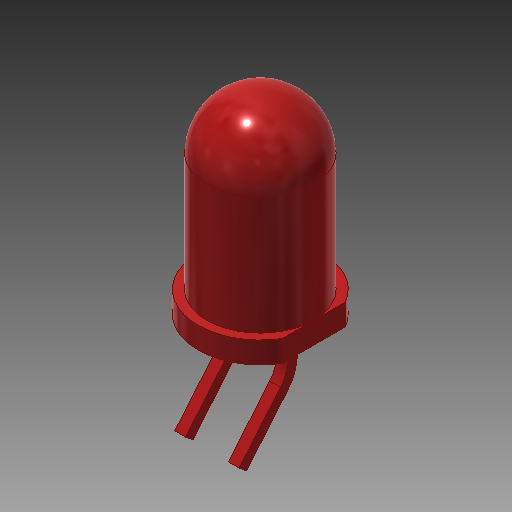
# Autodesk Inventor part: LED 5mm
Saved by Autodesk Inventor 2019.1 (Build 231200000, 200)
## iProperties
Created: 2012-08-15
Part Number: LED 5mm
Material: PC/ABS-Kunststoff
Document SubType Name: Modeling
Designer: rYan
Density: 1.493 g/cm^3
Mass: 0.251814 g
Surface Area: 1.94955 cm^2
Volume: 0.168663 cm^3
Appearance: Hellrot
Author: rYan
Autodesk Inventor part; units mm, degrees
note: some values were not read from the file. Chosen so that the rebuilt part matches the saved one: bend side of "Biegungsteil1".
ref_plane "XZ Plane" through (0, 0, 0) normal (0, 1, 0) x (-1, 0, 0)
ref_plane "XY Plane" through (0, 0, 0) normal (0, 0, 1) x (1, 0, 0)
sketch "Skizze1" plane through (0, 0, 0) normal (0, 1, 0) x (-1, 0, 0)
  line L0 (0, 0) -> (0, 9)
  line L1 (0, 0) -> (2.9, 0)
  line L2 (2.9, 0) -> (2.9, 1)
  line L3 (2.9, 1) -> (2.5, 1)
  line L4 (2.5, 1) -> (2.5, 6.5)
  arc A0 (2.5, 6.5) -> (0, 9) centre (0, 6.5) ccw
  dimension "d0" = 5.8
  dimension "d2" = 5
  dimension "d3" = 9
  dimension "d4" = 1
  constraints: 10 end point, 2 parallel, 2 perpendicular, 2 point on circle, 1 centre point, 1 point on line, 1 tangent, 1 vertical
  measures "d0" diameter of L2 L0
  measures "d2" diameter of L4 L0
  measures "d3" distance of L0.start L0.end
  measures "d4" distance of L1.end L2.end
revolve "Umdrehung1" add sketch "Skizze1" angle 360 about axis through (0, 0, 0) along (0, 0, 1)
ref_plane "Arbeitsebene2" through (2.5, 0, 3.75) normal (1, 0, 0) x (0, 1, 0)
sketch "Skizze2" plane through (2.5, 0, 3.75) normal (1, 0, 0) x (0, 1, 0)
  line L0 (-2.9, -3.75) -> (2.9, -3.75) projected
  line L1 (-2.9, -2.75) -> (2.9, -2.75) projected
  line L2 (-2.9, -2.75) -> (2.9, -2.75)
  line L3 (2.9, -2.75) -> (2.9, -3.75)
  line L4 (2.9, -3.75) -> (-2.9, -3.75)
  line L5 (-2.9, -3.75) -> (-2.9, -2.75)
  point P0 (0, -3.75)
  constraints: 8 end point, 2 parallel, 1 horizontal, 1 perpendicular
extrude "Extrusion1" cut sketch "Skizze2" along normal blind 1
sketch "Skizze3" plane through (0, 0, 0) normal (0, 0, -1) x (-1, 0, 0)
  line L0 (-1.5, 0.225) -> (-1, 0.225)
  line L1 (-1, 0.225) -> (-1, -0.225)
  line L2 (-1, -0.225) -> (-1.5, -0.225)
  line L3 (-1.5, -0.225) -> (-1.5, 0.225)
  line L4 (1, 0.225) -> (1.5, 0.225)
  line L5 (1.5, 0.225) -> (1.5, -0.225)
  line L6 (1.5, -0.225) -> (1, -0.225)
  line L7 (1, -0.225) -> (1, 0.225)
  line L8 (0, -4.06) -> (0, 4.06) projected
  line L9 (-3.58, 0) -> (3.98, 0) projected
  point P0 (0, 0)
  dimension "d8" = 0.5
  dimension "d10" = 0.45
  dimension "d11" = 3
  constraints: 16 end point, 4 parallel, 2 horizontal, 2 perpendicular, 5 other
  measures "d8" distance of L0.start L0.end
  measures "d10" distance of L0.end L1.end
  measures "d11" distance between parallel lines of L5 L3
extrude "Extrusion2" add sketch "Skizze3" along normal blind 5
sketch "Skizze4" plane through (1, -0.225, 0) normal (0, -1, 0) x (1, 0, 0)
  line L0 (1.4937, -1) -> (-4.2917, -1)
  line L1 (-3.9, 0) -> (1.5, 0) projected
  point P0 (-1, 0)
  dimension "d14" = 1
  constraints: 2 end point, 1 horizontal
  measures "d14" distance between parallel lines of L0 L1
bend part "Biegungsteil1" radius 1.4324 angle 40 line through (2.4937, -0.225, -1) along (-1, 0, 0) centre toward (0, -1, 0) moving side (0, 0, -1) both sides no
